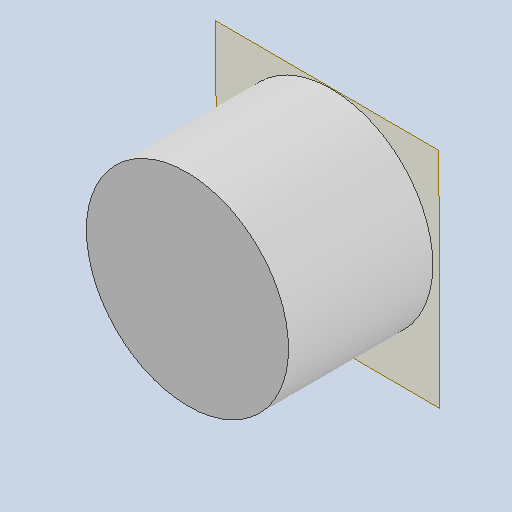
# Autodesk Inventor part: Motor
Saved by Autodesk Inventor 2026 (Build 300175050, 175E)
## iProperties
Created: 2025-08-03
Part Number: Motor
Material: Generic
Document SubType Name: Modeling
Designer: Cupri
Mass: 535 g
Surface Area: 249.815 cm^2
Volume: 297.029 cm^3
Density: 1.80117 g/cm^3
Appearance: Default
Author: Cupri
Autodesk Inventor part; units mm, degrees
ref_plane "YZ Plane" through (0, 0, 0) normal (1, 0, 0) x (0, 1, 0)
ref_plane "XZ Plane" through (0, 0, 0) normal (0, 1, 0) x (-1, 0, 0)
ref_plane "XY Plane" through (0, 0, 0) normal (0, 0, 1) x (1, 0, 0)
ref_plane "Work Plane1" through (-1.6314, -3.8779, 0.1345) normal (-0.0036, -0.0045, 1) x (1, 0, 0.0036)
sketch "Sketch1" plane through (-1.6314, -3.8779, 0.1345) normal (-0.0036, -0.0045, 1) x (1, 0, 0.0036)
  circle A0 centre (1.6309, 3.8772) radius 40.55
  dimension "d0" = 81.1
  constraints: 1 centre point, 1 coincident
  measures "d0" diameter of A0
extrude "Extrusion1" add sketch "Sketch1" along normal blind 57.5
body "Solid1"
